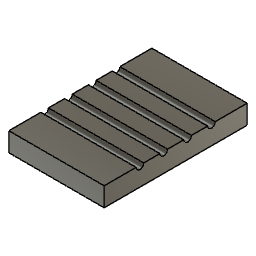
gabarito para solda das fitas leds (Autodesk Fusion 360 design; units mm, degrees)
Autodesk Fusion 360 part; units mm, degrees
note: some values were not read from the file. Set by a fixed rule: which sketch regions a step uses.
sketch "Sketch1" plane through (0, 0, 0) normal (0, 0, 1) x (1, 0, 0)
  line L0 (5, 7.5) -> (-5, 7.5)
  line L1 (-5, 7.5) -> (-5, -7.5)
  line L2 (-5, -7.5) -> (5, -7.5)
  line L3 (5, -7.5) -> (5, 7.5)
  line L4 (5, 7.5) -> (-5, -7.5) construction
  line L5 (-5, 7.5) -> (5, -7.5) construction
  dimension "d1" = 10
  dimension "d2" = 15
  constraint horizontal L0
  constraint perpendicular L0 L1
  constraint parallel L0 L2
  constraint parallel L1 L3
  constraint coincident L4 origin
  constraint coincident L5 origin
  measures "d1" distance of L1.end L2.end
  measures "d2" distance of L0.end L1.end
extrude "Extrude1" add sketch "Sketch1" along normal blind 3
sketch "Sketch2" plane through (5, 0, 0) normal (1, 0, 0) x (0, 1, 0)
  line L0 (-7.5, 0) -> (7.5, 0)
  line L1 (7.5, 0) -> (7.5, 3)
  line L2 (7.5, 3) -> (-7.5, 3)
  line L3 (-7.5, 3) -> (-7.5, 0)
  line L4 (0, 3) -> (5, 3) construction
  line L5 (5, 3) -> (3.75, 3) construction
  circle A0 centre (3.75, 3) radius 0.4
  line L6 (3.75, 3) -> (1.25, 3) construction
  circle A1 centre (1.25, 3) radius 0.4
  line L7 (0, 3) -> (0, 3.8715) construction
  circle A2 centre (-3.75, 3) radius 0.4
  circle A3 centre (-1.25, 3) radius 0.4
  dimension "d5" = 5
  dimension "d6" = 1.25
  dimension "d7" = 0.8
  dimension "d8" = 2.5
  dimension "d9" = 0.8
  constraint midpoint L2 L4.start
  constraint parallel L2 L4
  constraint parallel L2 L5
  constraint coincident L5.end A0.centre
  constraint parallel L4 L6
  constraint coincident L6.end A1.centre
  constraint perpendicular L2 L7
  constraint symmetric A0 L7 A2
  constraint symmetric A1 L7 A3
  measures "d5" distance of L4.start L4.end
  measures "d6" distance of L4.end L5.end
  measures "d7" diameter of A0
  measures "d8" distance of L5.end L6.end
  measures "d9" diameter of A1
extrude "Extrude2" cut sketch "Sketch2" against normal blind 15 contours L2 A2 | L2 A0 | L2 A3 | L2 A1 picked at (-3.8463, 2.8894) picked at (3.8833, 2.7915) picked at (-1.1781, 2.8008) picked at (1.1833, 2.8845)
extrude "Extrude3" cut 1 faces at (-1.6667, 2.5, 0) along direction (0, 0, 1) blind 1
